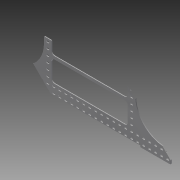
# Autodesk Inventor part: Strength Plate 2 (0.125 Steel)
Saved by Autodesk Inventor 2014 (Build 180170000, 170)
## iProperties
Created: 2014-02-11
Part Number: Strength Plate 2 (0.125 Steel)
Material: Steel
Document SubType Name: Modeling
Designer: Andrew Toennies
Mass: 1207.84 g
Surface Area: 1146.26 cm^2
Volume: 153.865 cm^3
Density: 7.85 g/cm^3
Appearance: Steel
Author: Andrew Toennies
Autodesk Inventor part; units mm, degrees
ref_plane "YZ Plane" through (0, 0, 0) normal (1, 0, 0) x (0, 1, 0)
ref_plane "XZ Plane" through (0, 0, 0) normal (0, 1, 0) x (-1, 0, 0)
ref_plane "XY Plane" through (0, 0, 0) normal (0, 0, 1) x (1, 0, 0)
sketch "Sketch1" plane through (0, 0, 0) normal (0, 0, 1) x (1, 0, 0)
  line L0 (0, 0) -> (0, 50.8)
  line L1 (0, 0) -> (688.975, 0)
  line L2 (688.975, 0) -> (688.975, 50.8)
  line L3 (150.8125, 50.8) -> (150.8125, 203.2)
  line L4 (150.8125, 203.2) -> (182.5625, 203.2)
  line L5 (182.5625, 203.2) -> (182.5625, 152.4)
  line L6 (182.5625, 152.4) -> (506.4125, 152.4)
  line L7 (506.4125, 152.4) -> (506.4125, 203.2)
  line L8 (506.4125, 203.2) -> (538.1625, 203.2)
  line L9 (538.1625, 203.2) -> (538.1625, 50.8)
  line L10 (538.1625, 50.8) -> (688.975, 50.8)
  line L11 (150.8125, 50.8) -> (0, 50.8)
  line L12 (182.5625, 127) -> (506.4125, 127)
  line L13 (506.4125, 127) -> (506.4125, 50.8)
  line L14 (506.4125, 50.8) -> (182.5625, 50.8)
  line L15 (182.5625, 50.8) -> (182.5625, 127)
  line L16 (163.5125, 190.5) -> (169.8625, 190.5) construction
  line L17 (163.5125, 187.1218) -> (169.8625, 187.1218)
  line L18 (169.8625, 193.8782) -> (163.5125, 193.8782)
  arc A0 (163.5125, 193.8782) -> (163.5125, 187.1218) centre (163.5125, 190.5) ccw
  arc A1 (169.8625, 187.1218) -> (169.8625, 193.8782) centre (169.8625, 190.5) ccw
  line L19 (163.5125, 165.1) -> (169.8625, 165.1) construction
  line L20 (163.5125, 161.7218) -> (169.8625, 161.7218)
  line L21 (169.8625, 168.4782) -> (163.5125, 168.4782)
  arc A2 (163.5125, 168.4782) -> (163.5125, 161.7218) centre (163.5125, 165.1) ccw
  arc A3 (169.8625, 161.7218) -> (169.8625, 168.4782) centre (169.8625, 165.1) ccw
  line L22 (163.5125, 139.7) -> (169.8625, 139.7) construction
  line L23 (163.5125, 136.3218) -> (169.8625, 136.3218)
  line L24 (169.8625, 143.0782) -> (163.5125, 143.0782)
  arc A4 (163.5125, 143.0782) -> (163.5125, 136.3218) centre (163.5125, 139.7) ccw
  arc A5 (169.8625, 136.3218) -> (169.8625, 143.0782) centre (169.8625, 139.7) ccw
  line L25 (163.5125, 114.3) -> (169.8625, 114.3) construction
  line L26 (163.5125, 110.9218) -> (169.8625, 110.9218)
  line L27 (169.8625, 117.6782) -> (163.5125, 117.6782)
  arc A6 (163.5125, 117.6782) -> (163.5125, 110.9218) centre (163.5125, 114.3) ccw
  arc A7 (169.8625, 110.9218) -> (169.8625, 117.6782) centre (169.8625, 114.3) ccw
  line L28 (163.5125, 88.9) -> (169.8625, 88.9) construction
  line L29 (163.5125, 85.5218) -> (169.8625, 85.5218)
  line L30 (169.8625, 92.2782) -> (163.5125, 92.2782)
  arc A8 (163.5125, 92.2782) -> (163.5125, 85.5218) centre (163.5125, 88.9) ccw
  arc A9 (169.8625, 85.5218) -> (169.8625, 92.2782) centre (169.8625, 88.9) ccw
  line L31 (163.5125, 63.5) -> (169.8625, 63.5) construction
  line L32 (163.5125, 60.1218) -> (169.8625, 60.1218)
  line L33 (169.8625, 66.8782) -> (163.5125, 66.8782)
  arc A10 (163.5125, 66.8782) -> (163.5125, 60.1218) centre (163.5125, 63.5) ccw
  arc A11 (169.8625, 60.1218) -> (169.8625, 66.8782) centre (169.8625, 63.5) ccw
  line L34 (163.5125, 38.1) -> (169.8625, 38.1) construction
  line L35 (163.5125, 34.7218) -> (169.8625, 34.7218)
  line L36 (169.8625, 41.4782) -> (163.5125, 41.4782)
  arc A12 (163.5125, 41.4782) -> (163.5125, 34.7218) centre (163.5125, 38.1) ccw
  arc A13 (169.8625, 34.7218) -> (169.8625, 41.4782) centre (169.8625, 38.1) ccw
  line L37 (163.5125, 12.7) -> (169.8625, 12.7) construction
  line L38 (163.5125, 9.3218) -> (169.8625, 9.3218)
  line L39 (169.8625, 16.0782) -> (163.5125, 16.0782)
  arc A14 (163.5125, 16.0782) -> (163.5125, 9.3218) centre (163.5125, 12.7) ccw
  arc A15 (169.8625, 9.3218) -> (169.8625, 16.0782) centre (169.8625, 12.7) ccw
  line L40 (344.4875, 207.962) -> (344.4875, 96.459) construction
  line L41 (525.4625, 190.5) -> (519.1125, 190.5) construction
  line L42 (525.4625, 187.1218) -> (519.1125, 187.1218)
  line L43 (519.1125, 193.8782) -> (525.4625, 193.8782)
  arc A16 (525.4625, 187.1218) -> (525.4625, 193.8782) centre (525.4625, 190.5) ccw
  arc A17 (519.1125, 193.8782) -> (519.1125, 187.1218) centre (519.1125, 190.5) ccw
  arc A18 (519.1125, 168.4782) -> (519.1125, 161.7218) centre (519.1125, 165.1) ccw
  line L44 (525.4625, 165.1) -> (519.1125, 165.1) construction
  line L45 (525.4625, 161.7218) -> (519.1125, 161.7218)
  line L46 (519.1125, 168.4782) -> (525.4625, 168.4782)
  arc A19 (525.4625, 161.7218) -> (525.4625, 168.4782) centre (525.4625, 165.1) ccw
  arc A20 (519.1125, 143.0782) -> (519.1125, 136.3218) centre (519.1125, 139.7) ccw
  line L47 (525.4625, 139.7) -> (519.1125, 139.7) construction
  line L48 (525.4625, 136.3218) -> (519.1125, 136.3218)
  line L49 (519.1125, 143.0782) -> (525.4625, 143.0782)
  arc A21 (525.4625, 136.3218) -> (525.4625, 143.0782) centre (525.4625, 139.7) ccw
  arc A22 (519.1125, 117.6782) -> (519.1125, 110.9218) centre (519.1125, 114.3) ccw
  line L50 (525.4625, 114.3) -> (519.1125, 114.3) construction
  line L51 (525.4625, 110.9218) -> (519.1125, 110.9218)
  line L52 (519.1125, 117.6782) -> (525.4625, 117.6782)
  arc A23 (525.4625, 110.9218) -> (525.4625, 117.6782) centre (525.4625, 114.3) ccw
  arc A24 (519.1125, 92.2782) -> (519.1125, 85.5218) centre (519.1125, 88.9) ccw
  line L53 (525.4625, 88.9) -> (519.1125, 88.9) construction
  line L54 (525.4625, 85.5218) -> (519.1125, 85.5218)
  line L55 (519.1125, 92.2782) -> (525.4625, 92.2782)
  arc A25 (525.4625, 85.5218) -> (525.4625, 92.2782) centre (525.4625, 88.9) ccw
  arc A26 (519.1125, 66.8782) -> (519.1125, 60.1218) centre (519.1125, 63.5) ccw
  line L56 (525.4625, 63.5) -> (519.1125, 63.5) construction
  line L57 (525.4625, 60.1218) -> (519.1125, 60.1218)
  line L58 (519.1125, 66.8782) -> (525.4625, 66.8782)
  arc A27 (525.4625, 60.1218) -> (525.4625, 66.8782) centre (525.4625, 63.5) ccw
  arc A28 (519.1125, 41.4782) -> (519.1125, 34.7218) centre (519.1125, 38.1) ccw
  line L59 (525.4625, 38.1) -> (519.1125, 38.1) construction
  line L60 (525.4625, 34.7218) -> (519.1125, 34.7218)
  line L61 (519.1125, 41.4782) -> (525.4625, 41.4782)
  arc A29 (525.4625, 34.7218) -> (525.4625, 41.4782) centre (525.4625, 38.1) ccw
  arc A30 (519.1125, 16.0782) -> (519.1125, 9.3218) centre (519.1125, 12.7) ccw
  line L62 (525.4625, 12.7) -> (519.1125, 12.7) construction
  line L63 (525.4625, 9.3218) -> (519.1125, 9.3218)
  line L64 (519.1125, 16.0782) -> (525.4625, 16.0782)
  arc A31 (525.4625, 9.3218) -> (525.4625, 16.0782) centre (525.4625, 12.7) ccw
  line L65 (493.7125, 143.0782) -> (500.0625, 143.0782)
  line L66 (500.0625, 139.7) -> (493.7125, 139.7) construction
  arc A32 (500.0625, 136.3218) -> (500.0625, 143.0782) centre (500.0625, 139.7) ccw
  arc A33 (493.7125, 143.0782) -> (493.7125, 136.3218) centre (493.7125, 139.7) ccw
  line L67 (500.0625, 136.3218) -> (493.7125, 136.3218)
  line L68 (468.3125, 143.0782) -> (474.6625, 143.0782)
  line L69 (474.6625, 139.7) -> (468.3125, 139.7) construction
  arc A34 (474.6625, 136.3218) -> (474.6625, 143.0782) centre (474.6625, 139.7) ccw
  arc A35 (468.3125, 143.0782) -> (468.3125, 136.3218) centre (468.3125, 139.7) ccw
  line L70 (474.6625, 136.3218) -> (468.3125, 136.3218)
  line L71 (442.9125, 143.0782) -> (449.2625, 143.0782)
  line L72 (449.2625, 139.7) -> (442.9125, 139.7) construction
  arc A36 (449.2625, 136.3218) -> (449.2625, 143.0782) centre (449.2625, 139.7) ccw
  arc A37 (442.9125, 143.0782) -> (442.9125, 136.3218) centre (442.9125, 139.7) ccw
  line L73 (449.2625, 136.3218) -> (442.9125, 136.3218)
  line L74 (417.5125, 143.0782) -> (423.8625, 143.0782)
  line L75 (423.8625, 139.7) -> (417.5125, 139.7) construction
  arc A38 (423.8625, 136.3218) -> (423.8625, 143.0782) centre (423.8625, 139.7) ccw
  arc A39 (417.5125, 143.0782) -> (417.5125, 136.3218) centre (417.5125, 139.7) ccw
  line L76 (423.8625, 136.3218) -> (417.5125, 136.3218)
  line L77 (392.1125, 143.0782) -> (398.4625, 143.0782)
  line L78 (398.4625, 139.7) -> (392.1125, 139.7) construction
  arc A40 (398.4625, 136.3218) -> (398.4625, 143.0782) centre (398.4625, 139.7) ccw
  arc A41 (392.1125, 143.0782) -> (392.1125, 136.3218) centre (392.1125, 139.7) ccw
  line L79 (398.4625, 136.3218) -> (392.1125, 136.3218)
  line L80 (366.7125, 143.0782) -> (373.0625, 143.0782)
  line L81 (373.0625, 139.7) -> (366.7125, 139.7) construction
  arc A42 (373.0625, 136.3218) -> (373.0625, 143.0782) centre (373.0625, 139.7) ccw
  arc A43 (366.7125, 143.0782) -> (366.7125, 136.3218) centre (366.7125, 139.7) ccw
  line L82 (373.0625, 136.3218) -> (366.7125, 136.3218)
  line L83 (341.3125, 143.0782) -> (347.6625, 143.0782)
  line L84 (347.6625, 139.7) -> (341.3125, 139.7) construction
  arc A44 (347.6625, 136.3218) -> (347.6625, 143.0782) centre (347.6625, 139.7) ccw
  arc A45 (341.3125, 143.0782) -> (341.3125, 136.3218) centre (341.3125, 139.7) ccw
  line L85 (347.6625, 136.3218) -> (341.3125, 136.3218)
  line L86 (315.9125, 143.0782) -> (322.2625, 143.0782)
  line L87 (322.2625, 139.7) -> (315.9125, 139.7) construction
  arc A46 (322.2625, 136.3218) -> (322.2625, 143.0782) centre (322.2625, 139.7) ccw
  arc A47 (315.9125, 143.0782) -> (315.9125, 136.3218) centre (315.9125, 139.7) ccw
  line L88 (322.2625, 136.3218) -> (315.9125, 136.3218)
  line L89 (290.5125, 143.0782) -> (296.8625, 143.0782)
  line L90 (296.8625, 139.7) -> (290.5125, 139.7) construction
  arc A48 (296.8625, 136.3218) -> (296.8625, 143.0782) centre (296.8625, 139.7) ccw
  arc A49 (290.5125, 143.0782) -> (290.5125, 136.3218) centre (290.5125, 139.7) ccw
  line L91 (296.8625, 136.3218) -> (290.5125, 136.3218)
  line L92 (265.1125, 143.0782) -> (271.4625, 143.0782)
  line L93 (271.4625, 139.7) -> (265.1125, 139.7) construction
  arc A50 (271.4625, 136.3218) -> (271.4625, 143.0782) centre (271.4625, 139.7) ccw
  arc A51 (265.1125, 143.0782) -> (265.1125, 136.3218) centre (265.1125, 139.7) ccw
  line L94 (271.4625, 136.3218) -> (265.1125, 136.3218)
  line L95 (239.7125, 143.0782) -> (246.0625, 143.0782)
  line L96 (246.0625, 139.7) -> (239.7125, 139.7) construction
  arc A52 (246.0625, 136.3218) -> (246.0625, 143.0782) centre (246.0625, 139.7) ccw
  arc A53 (239.7125, 143.0782) -> (239.7125, 136.3218) centre (239.7125, 139.7) ccw
  line L97 (246.0625, 136.3218) -> (239.7125, 136.3218)
  line L98 (214.3125, 143.0782) -> (220.6625, 143.0782)
  line L99 (220.6625, 139.7) -> (214.3125, 139.7) construction
  arc A54 (220.6625, 136.3218) -> (220.6625, 143.0782) centre (220.6625, 139.7) ccw
  arc A55 (214.3125, 143.0782) -> (214.3125, 136.3218) centre (214.3125, 139.7) ccw
  line L100 (220.6625, 136.3218) -> (214.3125, 136.3218)
  line L101 (188.9125, 143.0782) -> (195.2625, 143.0782)
  line L102 (195.2625, 139.7) -> (188.9125, 139.7) construction
  arc A56 (195.2625, 136.3218) -> (195.2625, 143.0782) centre (195.2625, 139.7) ccw
  arc A57 (188.9125, 143.0782) -> (188.9125, 136.3218) centre (188.9125, 139.7) ccw
  line L103 (195.2625, 136.3218) -> (188.9125, 136.3218)
  line L104 (544.5125, 41.4782) -> (550.8625, 41.4782)
  line L105 (550.8625, 38.1) -> (544.5125, 38.1) construction
  arc A58 (550.8625, 34.7218) -> (550.8625, 41.4782) centre (550.8625, 38.1) ccw
  arc A59 (544.5125, 41.4782) -> (544.5125, 34.7218) centre (544.5125, 38.1) ccw
  line L106 (550.8625, 34.7218) -> (544.5125, 34.7218)
  line L107 (544.5125, 16.0782) -> (550.8625, 16.0782)
  line L108 (550.8625, 12.7) -> (544.5125, 12.7) construction
  arc A60 (550.8625, 9.3218) -> (550.8625, 16.0782) centre (550.8625, 12.7) ccw
  line L109 (550.8625, 9.3218) -> (544.5125, 9.3218)
  arc A61 (544.5125, 16.0782) -> (544.5125, 9.3218) centre (544.5125, 12.7) ccw
  line L110 (569.9125, 41.4782) -> (576.2625, 41.4782)
  line L111 (576.2625, 38.1) -> (569.9125, 38.1) construction
  arc A62 (576.2625, 34.7218) -> (576.2625, 41.4782) centre (576.2625, 38.1) ccw
  arc A63 (569.9125, 41.4782) -> (569.9125, 34.7218) centre (569.9125, 38.1) ccw
  line L112 (576.2625, 34.7218) -> (569.9125, 34.7218)
  line L113 (569.9125, 16.0782) -> (576.2625, 16.0782)
  line L114 (576.2625, 12.7) -> (569.9125, 12.7) construction
  arc A64 (576.2625, 9.3218) -> (576.2625, 16.0782) centre (576.2625, 12.7) ccw
  line L115 (576.2625, 9.3218) -> (569.9125, 9.3218)
  arc A65 (569.9125, 16.0782) -> (569.9125, 9.3218) centre (569.9125, 12.7) ccw
  line L116 (595.3125, 41.4782) -> (601.6625, 41.4782)
  line L117 (601.6625, 38.1) -> (595.3125, 38.1) construction
  arc A66 (601.6625, 34.7218) -> (601.6625, 41.4782) centre (601.6625, 38.1) ccw
  arc A67 (595.3125, 41.4782) -> (595.3125, 34.7218) centre (595.3125, 38.1) ccw
  line L118 (601.6625, 34.7218) -> (595.3125, 34.7218)
  line L119 (595.3125, 16.0782) -> (601.6625, 16.0782)
  line L120 (601.6625, 12.7) -> (595.3125, 12.7) construction
  arc A68 (601.6625, 9.3218) -> (601.6625, 16.0782) centre (601.6625, 12.7) ccw
  line L121 (601.6625, 9.3218) -> (595.3125, 9.3218)
  arc A69 (595.3125, 16.0782) -> (595.3125, 9.3218) centre (595.3125, 12.7) ccw
  line L122 (620.7125, 41.4782) -> (627.0625, 41.4782)
  line L123 (627.0625, 38.1) -> (620.7125, 38.1) construction
  arc A70 (627.0625, 34.7218) -> (627.0625, 41.4782) centre (627.0625, 38.1) ccw
  arc A71 (620.7125, 41.4782) -> (620.7125, 34.7218) centre (620.7125, 38.1) ccw
  line L124 (627.0625, 34.7218) -> (620.7125, 34.7218)
  line L125 (620.7125, 16.0782) -> (627.0625, 16.0782)
  line L126 (627.0625, 12.7) -> (620.7125, 12.7) construction
  arc A72 (627.0625, 9.3218) -> (627.0625, 16.0782) centre (627.0625, 12.7) ccw
  line L127 (627.0625, 9.3218) -> (620.7125, 9.3218)
  arc A73 (620.7125, 16.0782) -> (620.7125, 9.3218) centre (620.7125, 12.7) ccw
  line L128 (646.1125, 41.4782) -> (652.4625, 41.4782)
  line L129 (652.4625, 38.1) -> (646.1125, 38.1) construction
  arc A74 (652.4625, 34.7218) -> (652.4625, 41.4782) centre (652.4625, 38.1) ccw
  arc A75 (646.1125, 41.4782) -> (646.1125, 34.7218) centre (646.1125, 38.1) ccw
  line L130 (652.4625, 34.7218) -> (646.1125, 34.7218)
  line L131 (646.1125, 16.0782) -> (652.4625, 16.0782)
  line L132 (652.4625, 12.7) -> (646.1125, 12.7) construction
  arc A76 (652.4625, 9.3218) -> (652.4625, 16.0782) centre (652.4625, 12.7) ccw
  line L133 (652.4625, 9.3218) -> (646.1125, 9.3218)
  arc A77 (646.1125, 16.0782) -> (646.1125, 9.3218) centre (646.1125, 12.7) ccw
  line L134 (671.5125, 41.4782) -> (677.8625, 41.4782)
  line L135 (677.8625, 38.1) -> (671.5125, 38.1) construction
  arc A78 (677.8625, 34.7218) -> (677.8625, 41.4782) centre (677.8625, 38.1) ccw
  arc A79 (671.5125, 41.4782) -> (671.5125, 34.7218) centre (671.5125, 38.1) ccw
  line L136 (677.8625, 34.7218) -> (671.5125, 34.7218)
  line L137 (671.5125, 16.0782) -> (677.8625, 16.0782)
  line L138 (677.8625, 12.7) -> (671.5125, 12.7) construction
  arc A80 (677.8625, 9.3218) -> (677.8625, 16.0782) centre (677.8625, 12.7) ccw
  line L139 (677.8625, 9.3218) -> (671.5125, 9.3218)
  arc A81 (671.5125, 16.0782) -> (671.5125, 9.3218) centre (671.5125, 12.7) ccw
  arc A82 (144.4625, 34.7218) -> (144.4625, 41.4782) centre (144.4625, 38.1) ccw
  line L140 (138.1125, 38.1) -> (144.4625, 38.1) construction
  line L141 (138.1125, 34.7218) -> (144.4625, 34.7218)
  line L142 (144.4625, 41.4782) -> (138.1125, 41.4782)
  arc A83 (138.1125, 41.4782) -> (138.1125, 34.7218) centre (138.1125, 38.1) ccw
  arc A84 (144.4625, 9.3218) -> (144.4625, 16.0782) centre (144.4625, 12.7) ccw
  line L143 (138.1125, 12.7) -> (144.4625, 12.7) construction
  line L144 (138.1125, 9.3218) -> (144.4625, 9.3218)
  line L145 (144.4625, 16.0782) -> (138.1125, 16.0782)
  arc A85 (138.1125, 16.0782) -> (138.1125, 9.3218) centre (138.1125, 12.7) ccw
  arc A86 (119.0625, 34.7218) -> (119.0625, 41.4782) centre (119.0625, 38.1) ccw
  line L146 (112.7125, 38.1) -> (119.0625, 38.1) construction
  line L147 (112.7125, 34.7218) -> (119.0625, 34.7218)
  line L148 (119.0625, 41.4782) -> (112.7125, 41.4782)
  arc A87 (112.7125, 41.4782) -> (112.7125, 34.7218) centre (112.7125, 38.1) ccw
  arc A88 (119.0625, 9.3218) -> (119.0625, 16.0782) centre (119.0625, 12.7) ccw
  line L149 (112.7125, 12.7) -> (119.0625, 12.7) construction
  line L150 (112.7125, 9.3218) -> (119.0625, 9.3218)
  line L151 (119.0625, 16.0782) -> (112.7125, 16.0782)
  arc A89 (112.7125, 16.0782) -> (112.7125, 9.3218) centre (112.7125, 12.7) ccw
  arc A90 (93.6625, 34.7218) -> (93.6625, 41.4782) centre (93.6625, 38.1) ccw
  line L152 (87.3125, 38.1) -> (93.6625, 38.1) construction
  line L153 (87.3125, 34.7218) -> (93.6625, 34.7218)
  line L154 (93.6625, 41.4782) -> (87.3125, 41.4782)
  arc A91 (87.3125, 41.4782) -> (87.3125, 34.7218) centre (87.3125, 38.1) ccw
  arc A92 (93.6625, 9.3218) -> (93.6625, 16.0782) centre (93.6625, 12.7) ccw
  line L155 (87.3125, 12.7) -> (93.6625, 12.7) construction
  line L156 (87.3125, 9.3218) -> (93.6625, 9.3218)
  line L157 (93.6625, 16.0782) -> (87.3125, 16.0782)
  arc A93 (87.3125, 16.0782) -> (87.3125, 9.3218) centre (87.3125, 12.7) ccw
  arc A94 (68.2625, 34.7218) -> (68.2625, 41.4782) centre (68.2625, 38.1) ccw
  line L158 (61.9125, 38.1) -> (68.2625, 38.1) construction
  line L159 (61.9125, 34.7218) -> (68.2625, 34.7218)
  line L160 (68.2625, 41.4782) -> (61.9125, 41.4782)
  arc A95 (61.9125, 41.4782) -> (61.9125, 34.7218) centre (61.9125, 38.1) ccw
  arc A96 (68.2625, 9.3218) -> (68.2625, 16.0782) centre (68.2625, 12.7) ccw
  line L161 (61.9125, 12.7) -> (68.2625, 12.7) construction
  line L162 (61.9125, 9.3218) -> (68.2625, 9.3218)
  line L163 (68.2625, 16.0782) -> (61.9125, 16.0782)
  arc A97 (61.9125, 16.0782) -> (61.9125, 9.3218) centre (61.9125, 12.7) ccw
  arc A98 (42.8625, 34.7218) -> (42.8625, 41.4782) centre (42.8625, 38.1) ccw
  line L164 (36.5125, 38.1) -> (42.8625, 38.1) construction
  line L165 (36.5125, 34.7218) -> (42.8625, 34.7218)
  line L166 (42.8625, 41.4782) -> (36.5125, 41.4782)
  arc A99 (36.5125, 41.4782) -> (36.5125, 34.7218) centre (36.5125, 38.1) ccw
  arc A100 (42.8625, 9.3218) -> (42.8625, 16.0782) centre (42.8625, 12.7) ccw
  line L167 (36.5125, 12.7) -> (42.8625, 12.7) construction
  line L168 (36.5125, 9.3218) -> (42.8625, 9.3218)
  line L169 (42.8625, 16.0782) -> (36.5125, 16.0782)
  arc A101 (36.5125, 16.0782) -> (36.5125, 9.3218) centre (36.5125, 12.7) ccw
  arc A102 (17.4625, 34.7218) -> (17.4625, 41.4782) centre (17.4625, 38.1) ccw
  line L170 (11.1125, 38.1) -> (17.4625, 38.1) construction
  line L171 (11.1125, 34.7218) -> (17.4625, 34.7218)
  line L172 (17.4625, 41.4782) -> (11.1125, 41.4782)
  arc A103 (11.1125, 41.4782) -> (11.1125, 34.7218) centre (11.1125, 38.1) ccw
  arc A104 (17.4625, 9.3218) -> (17.4625, 16.0782) centre (17.4625, 12.7) ccw
  line L173 (11.1125, 12.7) -> (17.4625, 12.7) construction
  line L174 (11.1125, 9.3218) -> (17.4625, 9.3218)
  line L175 (17.4625, 16.0782) -> (11.1125, 16.0782)
  arc A105 (11.1125, 16.0782) -> (11.1125, 9.3218) centre (11.1125, 12.7) ccw
  arc A106 (195.2625, 34.7218) -> (195.2625, 41.4782) centre (195.2625, 38.1) ccw
  line L176 (188.9125, 38.1) -> (195.2625, 38.1) construction
  line L177 (188.9125, 34.7218) -> (195.2625, 34.7218)
  line L178 (195.2625, 41.4782) -> (188.9125, 41.4782)
  arc A107 (188.9125, 41.4782) -> (188.9125, 34.7218) centre (188.9125, 38.1) ccw
  arc A108 (195.2625, 9.3218) -> (195.2625, 16.0782) centre (195.2625, 12.7) ccw
  line L179 (188.9125, 12.7) -> (195.2625, 12.7) construction
  line L180 (188.9125, 9.3218) -> (195.2625, 9.3218)
  line L181 (195.2625, 16.0782) -> (188.9125, 16.0782)
  arc A109 (188.9125, 16.0782) -> (188.9125, 9.3218) centre (188.9125, 12.7) ccw
  arc A110 (220.6625, 34.7218) -> (220.6625, 41.4782) centre (220.6625, 38.1) ccw
  line L182 (214.3125, 38.1) -> (220.6625, 38.1) construction
  line L183 (214.3125, 34.7218) -> (220.6625, 34.7218)
  line L184 (220.6625, 41.4782) -> (214.3125, 41.4782)
  arc A111 (214.3125, 41.4782) -> (214.3125, 34.7218) centre (214.3125, 38.1) ccw
  arc A112 (220.6625, 9.3218) -> (220.6625, 16.0782) centre (220.6625, 12.7) ccw
  line L185 (214.3125, 12.7) -> (220.6625, 12.7) construction
  line L186 (214.3125, 9.3218) -> (220.6625, 9.3218)
  line L187 (220.6625, 16.0782) -> (214.3125, 16.0782)
  arc A113 (214.3125, 16.0782) -> (214.3125, 9.3218) centre (214.3125, 12.7) ccw
  arc A114 (246.0625, 34.7218) -> (246.0625, 41.4782) centre (246.0625, 38.1) ccw
  line L188 (239.7125, 38.1) -> (246.0625, 38.1) construction
  line L189 (239.7125, 34.7218) -> (246.0625, 34.7218)
  line L190 (246.0625, 41.4782) -> (239.7125, 41.4782)
  arc A115 (239.7125, 41.4782) -> (239.7125, 34.7218) centre (239.7125, 38.1) ccw
  arc A116 (246.0625, 9.3218) -> (246.0625, 16.0782) centre (246.0625, 12.7) ccw
  line L191 (239.7125, 12.7) -> (246.0625, 12.7) construction
  line L192 (239.7125, 9.3218) -> (246.0625, 9.3218)
  line L193 (246.0625, 16.0782) -> (239.7125, 16.0782)
  arc A117 (239.7125, 16.0782) -> (239.7125, 9.3218) centre (239.7125, 12.7) ccw
  arc A118 (271.4625, 34.7218) -> (271.4625, 41.4782) centre (271.4625, 38.1) ccw
  line L194 (265.1125, 38.1) -> (271.4625, 38.1) construction
  line L195 (265.1125, 34.7218) -> (271.4625, 34.7218)
  line L196 (271.4625, 41.4782) -> (265.1125, 41.4782)
  arc A119 (265.1125, 41.4782) -> (265.1125, 34.7218) centre (265.1125, 38.1) ccw
  arc A120 (271.4625, 9.3218) -> (271.4625, 16.0782) centre (271.4625, 12.7) ccw
  line L197 (265.1125, 12.7) -> (271.4625, 12.7) construction
  line L198 (265.1125, 9.3218) -> (271.4625, 9.3218)
  line L199 (271.4625, 16.0782) -> (265.1125, 16.0782)
  arc A121 (265.1125, 16.0782) -> (265.1125, 9.3218) centre (265.1125, 12.7) ccw
  arc A122 (296.8625, 34.7218) -> (296.8625, 41.4782) centre (296.8625, 38.1) ccw
  line L200 (290.5125, 38.1) -> (296.8625, 38.1) construction
  line L201 (290.5125, 34.7218) -> (296.8625, 34.7218)
  line L202 (296.8625, 41.4782) -> (290.5125, 41.4782)
  arc A123 (290.5125, 41.4782) -> (290.5125, 34.7218) centre (290.5125, 38.1) ccw
  arc A124 (296.8625, 9.3218) -> (296.8625, 16.0782) centre (296.8625, 12.7) ccw
  line L203 (290.5125, 12.7) -> (296.8625, 12.7) construction
  line L204 (290.5125, 9.3218) -> (296.8625, 9.3218)
  line L205 (296.8625, 16.0782) -> (290.5125, 16.0782)
  arc A125 (290.5125, 16.0782) -> (290.5125, 9.3218) centre (290.5125, 12.7) ccw
  arc A126 (322.2625, 34.7218) -> (322.2625, 41.4782) centre (322.2625, 38.1) ccw
  line L206 (315.9125, 38.1) -> (322.2625, 38.1) construction
  line L207 (315.9125, 34.7218) -> (322.2625, 34.7218)
  line L208 (322.2625, 41.4782) -> (315.9125, 41.4782)
  arc A127 (315.9125, 41.4782) -> (315.9125, 34.7218) centre (315.9125, 38.1) ccw
  arc A128 (322.2625, 9.3218) -> (322.2625, 16.0782) centre (322.2625, 12.7) ccw
  line L209 (315.9125, 12.7) -> (322.2625, 12.7) construction
  line L210 (315.9125, 9.3218) -> (322.2625, 9.3218)
  line L211 (322.2625, 16.0782) -> (315.9125, 16.0782)
  arc A129 (315.9125, 16.0782) -> (315.9125, 9.3218) centre (315.9125, 12.7) ccw
  arc A130 (347.6625, 34.7218) -> (347.6625, 41.4782) centre (347.6625, 38.1) ccw
  line L212 (341.3125, 38.1) -> (347.6625, 38.1) construction
  line L213 (341.3125, 34.7218) -> (347.6625, 34.7218)
  line L214 (347.6625, 41.4782) -> (341.3125, 41.4782)
  arc A131 (341.3125, 41.4782) -> (341.3125, 34.7218) centre (341.3125, 38.1) ccw
  arc A132 (347.6625, 9.3218) -> (347.6625, 16.0782) centre (347.6625, 12.7) ccw
  line L215 (341.3125, 12.7) -> (347.6625, 12.7) construction
  line L216 (341.3125, 9.3218) -> (347.6625, 9.3218)
  line L217 (347.6625, 16.0782) -> (341.3125, 16.0782)
  arc A133 (341.3125, 16.0782) -> (341.3125, 9.3218) centre (341.3125, 12.7) ccw
  arc A134 (373.0625, 34.7218) -> (373.0625, 41.4782) centre (373.0625, 38.1) ccw
  line L218 (366.7125, 38.1) -> (373.0625, 38.1) construction
  line L219 (366.7125, 34.7218) -> (373.0625, 34.7218)
  line L220 (373.0625, 41.4782) -> (366.7125, 41.4782)
  arc A135 (366.7125, 41.4782) -> (366.7125, 34.7218) centre (366.7125, 38.1) ccw
  arc A136 (373.0625, 9.3218) -> (373.0625, 16.0782) centre (373.0625, 12.7) ccw
  line L221 (366.7125, 12.7) -> (373.0625, 12.7) construction
  line L222 (366.7125, 9.3218) -> (373.0625, 9.3218)
  line L223 (373.0625, 16.0782) -> (366.7125, 16.0782)
  arc A137 (366.7125, 16.0782) -> (366.7125, 9.3218) centre (366.7125, 12.7) ccw
  arc A138 (398.4625, 34.7218) -> (398.4625, 41.4782) centre (398.4625, 38.1) ccw
  line L224 (392.1125, 38.1) -> (398.4625, 38.1) construction
  line L225 (392.1125, 34.7218) -> (398.4625, 34.7218)
  line L226 (398.4625, 41.4782) -> (392.1125, 41.4782)
  arc A139 (392.1125, 41.4782) -> (392.1125, 34.7218) centre (392.1125, 38.1) ccw
  arc A140 (398.4625, 9.3218) -> (398.4625, 16.0782) centre (398.4625, 12.7) ccw
  line L227 (392.1125, 12.7) -> (398.4625, 12.7) construction
  line L228 (392.1125, 9.3218) -> (398.4625, 9.3218)
  line L229 (398.4625, 16.0782) -> (392.1125, 16.0782)
  arc A141 (392.1125, 16.0782) -> (392.1125, 9.3218) centre (392.1125, 12.7) ccw
  arc A142 (423.8625, 34.7218) -> (423.8625, 41.4782) centre (423.8625, 38.1) ccw
  line L230 (417.5125, 38.1) -> (423.8625, 38.1) construction
  line L231 (417.5125, 34.7218) -> (423.8625, 34.7218)
  line L232 (423.8625, 41.4782) -> (417.5125, 41.4782)
  arc A143 (417.5125, 41.4782) -> (417.5125, 34.7218) centre (417.5125, 38.1) ccw
  arc A144 (423.8625, 9.3218) -> (423.8625, 16.0782) centre (423.8625, 12.7) ccw
  line L233 (417.5125, 12.7) -> (423.8625, 12.7) construction
  line L234 (417.5125, 9.3218) -> (423.8625, 9.3218)
  line L235 (423.8625, 16.0782) -> (417.5125, 16.0782)
  arc A145 (417.5125, 16.0782) -> (417.5125, 9.3218) centre (417.5125, 12.7) ccw
  arc A146 (449.2625, 34.7218) -> (449.2625, 41.4782) centre (449.2625, 38.1) ccw
  line L236 (442.9125, 38.1) -> (449.2625, 38.1) construction
  line L237 (442.9125, 34.7218) -> (449.2625, 34.7218)
  line L238 (449.2625, 41.4782) -> (442.9125, 41.4782)
  arc A147 (442.9125, 41.4782) -> (442.9125, 34.7218) centre (442.9125, 38.1) ccw
  arc A148 (449.2625, 9.3218) -> (449.2625, 16.0782) centre (449.2625, 12.7) ccw
  line L239 (442.9125, 12.7) -> (449.2625, 12.7) construction
  line L240 (442.9125, 9.3218) -> (449.2625, 9.3218)
  line L241 (449.2625, 16.0782) -> (442.9125, 16.0782)
  arc A149 (442.9125, 16.0782) -> (442.9125, 9.3218) centre (442.9125, 12.7) ccw
  arc A150 (474.6625, 34.7218) -> (474.6625, 41.4782) centre (474.6625, 38.1) ccw
  line L242 (468.3125, 38.1) -> (474.6625, 38.1) construction
  line L243 (468.3125, 34.7218) -> (474.6625, 34.7218)
  line L244 (474.6625, 41.4782) -> (468.3125, 41.4782)
  arc A151 (468.3125, 41.4782) -> (468.3125, 34.7218) centre (468.3125, 38.1) ccw
  arc A152 (474.6625, 9.3218) -> (474.6625, 16.0782) centre (474.6625, 12.7) ccw
  line L245 (468.3125, 12.7) -> (474.6625, 12.7) construction
  line L246 (468.3125, 9.3218) -> (474.6625, 9.3218)
  line L247 (474.6625, 16.0782) -> (468.3125, 16.0782)
  arc A153 (468.3125, 16.0782) -> (468.3125, 9.3218) centre (468.3125, 12.7) ccw
  arc A154 (500.0625, 34.7218) -> (500.0625, 41.4782) centre (500.0625, 38.1) ccw
  line L248 (493.7125, 38.1) -> (500.0625, 38.1) construction
  line L249 (493.7125, 34.7218) -> (500.0625, 34.7218)
  line L250 (500.0625, 41.4782) -> (493.7125, 41.4782)
  arc A155 (493.7125, 41.4782) -> (493.7125, 34.7218) centre (493.7125, 38.1) ccw
  arc A156 (500.0625, 9.3218) -> (500.0625, 16.0782) centre (500.0625, 12.7) ccw
  line L251 (493.7125, 12.7) -> (500.0625, 12.7) construction
  line L252 (493.7125, 9.3218) -> (500.0625, 9.3218)
  line L253 (500.0625, 16.0782) -> (493.7125, 16.0782)
  arc A157 (493.7125, 16.0782) -> (493.7125, 9.3218) centre (493.7125, 12.7) ccw
  point P0 (166.6875, 190.5)
  point P1 (166.6875, 165.1)
  point P2 (166.6875, 139.7)
  point P3 (166.6875, 114.3)
  point P4 (166.6875, 88.9)
  point P5 (166.6875, 63.5)
  point P6 (166.6875, 38.1)
  point P7 (166.6875, 12.7)
  point P8 (522.2875, 190.5)
  point P9 (522.2875, 165.1)
  point P10 (522.2875, 139.7)
  point P11 (522.2875, 114.3)
  point P12 (522.2875, 88.9)
  point P13 (522.2875, 63.5)
  point P14 (522.2875, 38.1)
  point P15 (522.2875, 12.7)
  point P16 (496.8875, 139.7)
  point P17 (471.4875, 139.7)
  point P18 (446.0875, 139.7)
  point P19 (420.6875, 139.7)
  point P20 (395.2875, 139.7)
  point P21 (369.8875, 139.7)
  point P22 (344.4875, 139.7)
  point P23 (319.0875, 139.7)
  point P24 (293.6875, 139.7)
  point P25 (268.2875, 139.7)
  point P26 (242.8875, 139.7)
  point P27 (217.4875, 139.7)
  point P28 (192.0875, 139.7)
  point P29 (547.6875, 38.1)
  point P30 (547.6875, 12.7)
  point P31 (573.0875, 38.1)
  point P32 (573.0875, 12.7)
  point P33 (598.4875, 38.1)
  point P34 (598.4875, 12.7)
  point P35 (623.8875, 38.1)
  point P36 (623.8875, 12.7)
  point P37 (649.2875, 38.1)
  point P38 (649.2875, 12.7)
  point P39 (674.6875, 38.1)
  point P40 (674.6875, 12.7)
  point P41 (141.2875, 38.1)
  point P42 (141.2875, 12.7)
  point P43 (115.8875, 38.1)
  point P44 (115.8875, 12.7)
  point P45 (90.4875, 38.1)
  point P46 (90.4875, 12.7)
  point P47 (65.0875, 38.1)
  point P48 (65.0875, 12.7)
  point P49 (39.6875, 38.1)
  point P50 (39.6875, 12.7)
  point P51 (14.2875, 38.1)
  point P52 (14.2875, 12.7)
  point P53 (192.0875, 38.1)
  point P54 (192.0875, 12.7)
  point P55 (217.4875, 38.1)
  point P56 (217.4875, 12.7)
  point P57 (242.8875, 38.1)
  point P58 (242.8875, 12.7)
  point P59 (268.2875, 38.1)
  point P60 (268.2875, 12.7)
  point P61 (293.6875, 38.1)
  point P62 (293.6875, 12.7)
  point P63 (319.0875, 38.1)
  point P64 (319.0875, 12.7)
  point P65 (344.4875, 38.1)
  point P66 (344.4875, 12.7)
  point P67 (369.8875, 38.1)
  point P68 (369.8875, 12.7)
  point P69 (395.2875, 38.1)
  point P70 (395.2875, 12.7)
  point P71 (420.6875, 38.1)
  point P72 (420.6875, 12.7)
  point P73 (446.0875, 38.1)
  point P74 (446.0875, 12.7)
  point P75 (471.4875, 38.1)
  point P76 (471.4875, 12.7)
  point P77 (496.8875, 38.1)
  point P78 (496.8875, 12.7)
  dimension "d0" = 50.8
  dimension "d2" = 50.8
  dimension "d3" = 152.4
  dimension "d4" = 31.75
  dimension "d5" = 50.8
  dimension "d7" = 50.8
  dimension "d8" = 31.75
  dimension "d10" = 31.75
  dimension "d11" = 31.75
  dimension "d14" = 6.7564
  dimension "d16" = 12.7
  dimension "d17" = 6.35
  dimension "d32" = 166.6875
  dimension "d33" = 150.8125
  dimension "d34" = 150.8125
  dimension "d75" = 688.975
  dimension "d76" = 76.2
  dimension "d79" = 25.4
  dimension "d86" = 25.4
  dimension "d91" = 25.4
  dimension "d94" = 25.4
  dimension "d101" = 25.4
  dimension "d108" = 25.4
  constraints: 666 end point, 316 point on circle, 158 centre point, 56 symmetric about line, 10 parallel, 5 horizontal, 5 perpendicular, 4 tangent, 3 collinear, 2 vertical, 1 midpoint, 856 other
  measures "d0" distance of L0.start L0.end
  measures "d2" distance of L1.end L2.end
  measures "d3" distance of L3.start L3.end
  measures "d4" distance of L3.end L4.end
  measures "d5" distance of L4.end L5.end
  measures "d7" distance of L6.end L7.end
  measures "d8" distance of L7.end L8.end
  measures "d10" distance between parallel lines of L3 L15
  measures "d11" distance between parallel lines of L9 L13
  measures "d14" distance between parallel lines of L17 L18
  measures "d16" distance from line of L4 point (166.688, 190.5)
  measures "d17" distance of L16.start L16.end
  measures "d32" distance from line of L0 point (166.688, 190.5)
  measures "d33" distance between parallel lines of L0 L3
  measures "d34" distance between parallel lines of L2 L9
  measures "d75" distance between parallel lines of L0 L2
  measures "d76" distance between parallel lines of L14 L12
  measures "d79" distance of L17.end L20.end
  measures "d86" distance of L48.end L67.end
  measures "d91" distance of point (166.688, 139.7) point (192.087, 139.7)
  measures "d94" distance of L61.start L104.start
  measures "d101" distance of L36.start L142.start
  measures "d108" distance of L36.start L178.start
extrude "Extrusion2" add sketch "Sketch1" along normal blind 3.175 contours L0 L11 L3 L4 L5 L6 L7 L8 L9 L10 L2 L1 | L65 A32 L67 A33 | L68 A34 L70 A35 | L71 A36 L73 A37 | L74 A38 L76 A39 | L77 A40 L79 A41 | L80 A42 L82 A43 | L83 A44 L85 A45 | L86 A46 L88 A47 | L89 A48 L91 A49 | L92 A50 L94 A51 | L95 A52 L97 A53 | L98 A54 L100 A55 | L101 A56 L103 A57
fillet "Fillet4" radius 25.4 2 edges at (538.1625, 50.8, 1.5875) (150.8125, 50.8, 1.5875)
fillet "Fillet5" radius 3.175 8 edges at (538.1625, 203.2, 1.5875) (506.4125, 203.2, 1.5875) (150.8125, 203.2, 1.5875) (182.5625, 203.2, 1.5875) (0, 50.8, 1.5875) (0, 0, 1.5875) (688.975, 0, 1.5875) (688.975, 50.8, 1.5875)
fillet "Fillet6" radius 12.7 6 edges at (506.4125, 50.8, 1.5875) (182.5625, 50.8, 1.5875) (182.5625, 127, 1.5875) (182.5625, 152.4, 1.5875) (506.4125, 127, 1.5875) (506.4125, 152.4, 1.5875)
sketch "Sketch2" plane through (0, 0, 0) normal (0, 0, -1) x (-1, 0, 0)
  line L0 (-685.8, 0) -> (-3.175, 0) projected
  arc A0 (-493.7125, 127) -> (-506.4125, 114.3) centre (-493.7125, 114.3) ccw projected
  line L1 (-493.7125, 127) -> (-195.2625, 127) projected
  arc A1 (-182.5625, 114.3) -> (-195.2625, 127) centre (-195.2625, 114.3) ccw projected
  line L2 (-169.8625, 193.8782) -> (-163.5125, 193.8782) projected
  line L3 (-506.4125, 114.3) -> (-506.4125, 127)
  line L4 (-493.7125, 139.7) -> (-195.2625, 139.7)
  line L5 (-182.5625, 127) -> (-182.5625, 114.3)
  line L6 (-611.1875, 0) -> (-611.1875, 6.35)
  line L7 (-611.1875, 6.35) -> (-77.7875, 6.35)
  line L8 (-77.7875, 6.35) -> (-77.7875, 0)
  arc A2 (-493.7125, 139.7) -> (-506.4125, 127) centre (-493.7125, 127) ccw
  arc A3 (-182.5625, 127) -> (-195.2625, 139.7) centre (-195.2625, 127) ccw
  point P0 (0, 0)
  point P1 (-506.4125, 139.7)
  point P2 (-182.5625, 139.7)
  dimension "d118" = 25.4
  dimension "d119" = 323.85
  dimension "d120" = 6.35
  dimension "d121" = 533.4
  dimension "d122" = 77.7875
  dimension "d123" = 12.7
  constraints: 12 end point, 6 point on line, 5 tangent, 4 point on circle, 3 perpendicular, 2 centre point, 2 parallel, 1 equal radius
  measures "d118" distance of L3.start point (-506.413, 139.7)
  measures "d119" distance of point (-506.413, 139.7) point (-182.563, 139.7)
  measures "d120" distance of L6.start L6.end
  measures "d121" distance of L6.end L7.end
  measures "d122" distance of point (0, 0) L8.end
  measures "d123" radius of A2
extrude "Extrusion3" cut sketch "Sketch2" against normal blind 3.175
fillet "Fillet7" radius 3.175 4 edges at (77.7875, 6.35, 1.5875) (77.7875, 0, 1.5875) (611.1875, 6.35, 1.5875) (611.1875, 0, 1.5875)
body "Solid2"
